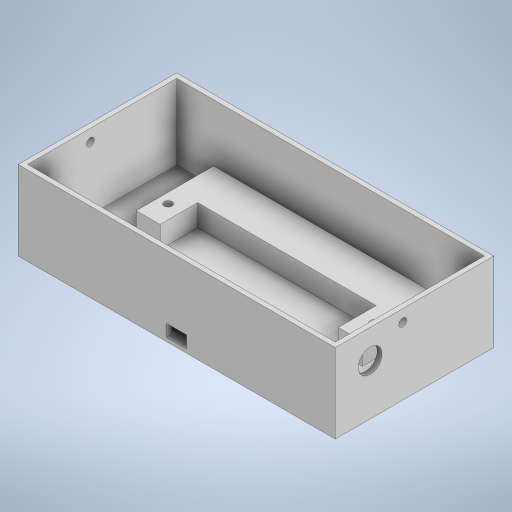
# Autodesk Inventor part: Konsole
Saved by Autodesk Inventor 2024 (Build 280153000, 153)
## iProperties
Created: 2024-03-10
Part Number: Konsole
Material: Generisch
Document SubType Name: Modeling
Designer: User
Density: 1 g/cm^3
Appearance: Vorgabe
Author: User
Autodesk Inventor part; units mm, degrees
ref_plane "YZ Plane" through (0, 0, 0) normal (1, 0, 0) x (0, 1, 0)
ref_plane "XZ Plane" through (0, 0, 0) normal (0, 1, 0) x (-1, 0, 0)
ref_plane "XY Plane" through (0, 0, 0) normal (0, 0, 1) x (1, 0, 0)
sketch "Skizze1" plane through (0, 0, 0) normal (0, 0, 1) x (1, 0, 0)
  line L0 (-25.5765, 16.0824) -> (54.4235, 16.0824)
  line L1 (54.4235, 16.0824) -> (54.4235, -23.9176)
  line L2 (54.4235, -23.9176) -> (-25.5765, -23.9176)
  line L3 (-25.5765, -23.9176) -> (-25.5765, 16.0824)
  line L4 (-24.3765, 14.8824) -> (53.2235, 14.8824)
  line L5 (53.2235, 14.8824) -> (53.2235, -22.7176)
  line L6 (53.2235, -22.7176) -> (-24.3765, -22.7176)
  line L7 (-24.3765, -22.7176) -> (-24.3765, 14.8824)
  point P0 (0, 0)
  dimension "d0" = 80
  dimension "d1" = 40
  dimension "d2" = 1.2
  dimension "d3" = 1.2
  dimension "d4" = 1.2
  dimension "d5" = 1.2
  constraints: 16 end point, 4 parallel, 2 horizontal, 2 perpendicular
  measures "d0" distance of L1.end L2.end
  measures "d1" distance of L0.end L1.end
  measures "d2" distance between parallel lines of L0 L4
  measures "d3" distance between parallel lines of L1 L5
  measures "d4" distance between parallel lines of L6 L2
  measures "d5" distance between parallel lines of L3 L7
extrude "Extrusion1" add sketch "Skizze1" along normal blind 1 contours L4 L5 L6 L7
extrude "Extrusion2" add sketch "Skizze1" along normal blind 20
sketch "Skizze2" plane through (0, 0, 1) normal (0, 0, 1) x (1, 0, 0)
  line L0 (-24.3765, 14.8824) -> (53.2235, 14.8824) projected
  line L1 (-21.8265, 14.8824) -> (50.6735, 14.8824)
  line L2 (50.6735, 14.8824) -> (50.6735, -5.6176)
  line L3 (50.6735, -5.6176) -> (-21.8265, -5.6176)
  line L4 (-21.8265, -5.6176) -> (-21.8265, 14.8824)
  line L5 (-24.3765, -22.7176) -> (-24.3765, 14.8824) projected
  line L6 (53.2235, 14.8824) -> (53.2235, -22.7176) projected
  line L7 (-14.0765, 13.8824) -> (42.9235, 13.8824)
  line L8 (42.9235, 13.8824) -> (42.9235, -6.1176)
  line L9 (42.9235, -6.1176) -> (-14.0765, -6.1176)
  line L10 (-14.0765, -6.1176) -> (-14.0765, 13.8824)
  line L11 (-8.0765, -6.1176) -> (36.9235, -6.1176)
  line L12 (36.9235, -6.1176) -> (36.9235, 3.8824)
  line L13 (36.9235, 3.8824) -> (-8.0765, 3.8824)
  line L14 (-8.0765, 3.8824) -> (-8.0765, -6.1176)
  circle A0 centre (40.3835, -0.1176) radius 1
  circle A1 centre (-11.5365, -0.1176) radius 1
  point P0 (0, 0)
  point P1 (-21.8265, 4.6324)
  point P2 (50.6735, 4.6324)
  point P3 (-14.0765, -5.6176)
  point P4 (-8.0765, -5.6176)
  point P5 (36.9235, -5.6176)
  point P6 (42.9235, -5.6176)
  dimension "d10" = 20.5
  dimension "d11" = 72.5
  dimension "d12" = 2.55
  dimension "d13" = 2.55
  dimension "d14" = 1
  dimension "d15" = 57
  dimension "d16" = 7.75
  dimension "d17" = 20
  dimension "d18" = 2
  dimension "d19" = 2
  dimension "d20" = 2.54
  dimension "d21" = 2.54
  dimension "d25" = 14
  dimension "d26" = 14
  dimension "d27" = 10
  dimension "d28" = 6
  dimension "d29" = 6
  constraints: 24 end point, 6 parallel, 3 horizontal, 3 perpendicular, 2 centre point, 2 midpoint, 2 point on line
  measures "d10" distance of L3.end L1.start
  measures "d11" distance of L2.end L3.end
  measures "d12" distance from line of L5 point (-21.826, 4.632)
  measures "d13" distance from line of L6 point (50.674, 4.632)
  measures "d14" distance between parallel lines of L0 L7
  measures "d15" distance of L8.end L9.end
  measures "d16" distance between parallel lines of L4 L10
  measures "d17" distance of L7.end L8.end
  measures "d18" diameter of A0
  measures "d19" diameter of A1
  measures "d20" distance from line of L10 A1.centre
  measures "d21" distance from line of L8 A0.centre
  measures "d25" distance from line of L7 A0.centre
  measures "d26" distance from line of L7 A1.centre
  measures "d27" distance between parallel lines of L9 L13
  measures "d28" distance between parallel lines of L10 L14
  measures "d29" distance between parallel lines of L8 L12
extrude "Extrusion3" add sketch "Skizze2" along normal blind 5.5 contours L10 L7 L8 L3 L12 L13 L14
sketch "Skizze3" plane through (54.4235, -23.9176, 0) normal (1, 0, 0) x (0, 0, -1)
  circle A0 centre (-17, 17) radius 1
  line L0 (0, 40) -> (-20, 40) projected
  line L1 (-20, 0) -> (-20, 40) projected
  circle A1 centre (-12.7552, 8.7755) radius 3
  point P0 (0, 23.9176)
  dimension "d32" = 2
  dimension "d33" = 23
  dimension "d34" = 3
  dimension "d35" = 6
  constraints: 2 centre point
  measures "d32" diameter of A0
  measures "d33" distance from line of L0 A0.centre
  measures "d34" distance from line of L1 A0.centre
  measures "d35" diameter of A1
extrude "Extrusion4" cut sketch "Skizze3" against normal through all contours A0
extrude "Extrusion5" cut sketch "Skizze3" against normal blind 1.2 contours A1
sketch "Skizze4" plane through (-25.5765, -23.9176, 0) normal (0, -1, 0) x (1, 0, 0)
  line L0 (78.8, 1) -> (1.2, 1) projected
  line L1 (37.5, 1) -> (42.5, 1)
  line L2 (42.5, 1) -> (42.5, 4)
  line L3 (42.5, 4) -> (37.5, 4)
  line L4 (37.5, 4) -> (37.5, 1)
  line L5 (0, 0) -> (0, 20) projected
  line L6 (80, 0) -> (80, 20) projected
  point P0 (25.5765, 0)
  point P1 (37.5, 2.5)
  point P2 (42.5, 2.5)
  dimension "d40" = 5
  dimension "d41" = 3
  dimension "d42" = 37.5
  dimension "d43" = 37.5
  constraints: 8 end point, 2 midpoint, 2 parallel, 1 horizontal, 1 perpendicular, 1 point on line
  measures "d40" distance of L3.end L2.end
  measures "d41" distance of L2.end L1.end
  measures "d42" distance from line of L5 point (37.5, 2.5)
  measures "d43" distance from line of L6 point (42.5, 2.5)
extrude "Extrusion6" cut sketch "Skizze4" against normal blind 1.2
